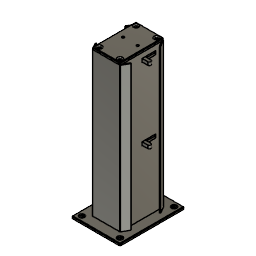
fpv dropper V1 (Autodesk Fusion 360 archive; units mm, degrees)
design "fpv dropper" references "SG90 - Micro Servo 9g - Tower Pro", "fpv dropper"
Autodesk Fusion 360 part; units mm, degrees
sketch "Sketch1" plane through (0, 0, 0) normal (0, 0, 1) x (1, 0, 0)
  line L0 (0, 0) -> (37, 0)
  line L1 (37, 0) -> (37, 52.5)
  line L2 (37, 52.5) -> (0, 52.5)
  line L3 (0, 52.5) -> (0, 0)
  line L4 (37, 52.5) -> (41.9497, 57.4497)
  line L5 (37, 52.5) -> (40, 52.5) construction
  line L6 (0, 0) -> (-4.9497, -4.9497)
  line L7 (0, 0) -> (3, 0) construction
  line L8 (-4.9497, -4.9497) -> (41.9497, -4.9497)
  line L9 (41.9497, -4.9497) -> (41.9497, 57.4497)
  line L10 (41.9497, 57.4497) -> (-4.9497, 57.4497)
  line L11 (-4.9497, 57.4497) -> (-4.9497, -4.9497)
  circle A0 centre (0, 0) radius 1.5
  circle A1 centre (37, 0) radius 1.5
  circle A2 centre (0, 52.5) radius 1.5
  circle A3 centre (37, 52.5) radius 1.5
  dimension "d1" = 37
  dimension "d2" = 52.5
  dimension "d3" = 7
  dimension "d4" = 45
  dimension "d5" = 135
  dimension "d6" = 7
  dimension "d7" = 3
  dimension "d10" = 37
  dimension "d11" = 52.5
  constraint horizontal L0
  constraint vertical L1
  constraint horizontal L2
  constraint vertical L3
  constraint coincident L0.start L3.end
  constraint horizontal L5
  constraint horizontal L7
  constraint horizontal L8
  constraint vertical L9
  constraint horizontal L10
  constraint vertical L11
  measures "d1" distance of L0.start L0.end
  measures "d2" distance of L0.start L2.end
  measures "d3" distance of L1.end L4.end
  measures "d4" angle of L4 L5
  measures "d5" angle of L6 L7
  measures "d6" distance of L0.start L6.end
  measures "d7" diameter of A0
extrude "Extrude1" add sketch "Sketch1" along normal blind 9 contours L0 L3 A0 | L3 L6 A0 | L0 L6 A0 | L0 L1 A1 | L0 L1 A1 | L2 L3 A2 | L2 L3 A2 | L1 L2 A3 | L1 L4 A3 | L2 L4 A3 makes body 1 at (-1.3822, 51.9173, 3) makes body 2 at (1.4925, -0.1494, 3) makes body 3 at (35.6827, 53.2174, 6) makes body 4 at (36.3157, 1.3348, 6)
extrude "Extrude2" add sketch "Sketch1" along normal blind 2 contours L0 L1 L2 L3 A0 A1 A2 A3 | L0 L1 L4 L6 L8 L9 A0 A1 A3 | L2 L3 L4 L6 L10 L11 A0 A2 A3 bodies 1 2 3 4
extrude "Extrude3" cut 4 faces at (-0.8158, 52.7169, 9) (37.3665, 53.1348, 9) (36.6279, -0.2656, 9) (-0.3779, 0.6986, 9) along direction (0, 0, -1) blind 28 on bodies 1 bodies 1
hole "Hole1" at (0, 0, 2) direction (0, 0, -1) diameter 3 depth 3 tip angle 118 counterbore diameter 5.1 counterbore depth 1 bodies 1
pattern_linear "R-Pattern1" count 2 spacing 52.5 along (0, 1, 0) count 2 spacing 37 along (1, 0, 0) of "Hole1"
sketch "Sketch2" plane through (0, 0, 2) normal (0, 0, 1) x (-1, 0, 0)
  circle A0 centre (-37, -52.5) radius 2.55
  circle A1 centre (-37, 0) radius 2.55
  circle A2 centre (0, -52.5) radius 2.55
  circle A3 centre (0, 0) radius 2.55
  line L0 (4.9497, -57.4497) -> (4.9497, 4.9497)
  line L1 (4.9497, 4.9497) -> (-41.9497, 4.9497)
  line L2 (-41.9497, 4.9497) -> (-41.9497, -57.4497)
  line L3 (-41.9497, -57.4497) -> (4.9497, -57.4497)
  line L4 (4.9497, -57.4497) -> (-41.9497, -57.4497)
  line L5 (-41.9497, -57.4497) -> (-41.9497, 4.9497)
  line L6 (-41.9497, 4.9497) -> (4.9497, 4.9497)
  line L7 (4.9497, 4.9497) -> (4.9497, -57.4497)
  line L8 (-31.9497, -5.0503) -> (-5.0503, -5.0503)
  line L9 (-5.0503, -5.0503) -> (-5.0503, -47.4497)
  line L10 (-5.0503, -47.4497) -> (-31.9497, -47.4497)
  line L11 (-31.9497, -47.4497) -> (-31.9497, -5.0503)
  line L12 (-29.9497, -7.0503) -> (-7.0503, -7.0503)
  line L13 (-7.0503, -7.0503) -> (-7.0503, -45.4497)
  line L14 (-7.0503, -45.4497) -> (-29.9497, -45.4497)
  line L15 (-29.9497, -45.4497) -> (-29.9497, -7.0503)
  dimension "d27" = 10
  dimension "d28" = 2
  constraint horizontal L4
  constraint vertical L5
  constraint horizontal L6
  constraint vertical L7
  constraint coincident L1.end L2.start
  constraint coincident L0.start L3.end
named bodies: "First Latch", "Tube Bot", "Forth Geneva", "Forth Latch", "Third Geneva", "Third Latch", "Second Geneva", "Second Latch", "First Geneva", "Tube Top", "Tube Mid", "Lid", "Shell"
